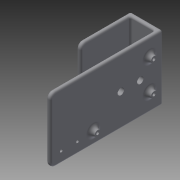
# Autodesk Inventor part: bed-stopper
Saved by Autodesk Inventor 2014 (Build 180170000, 170)
## iProperties
Created: 2017-07-21
Part Number: bed-stopper
Material: 一般
Document SubType Name: Modeling
Designer: hide
Density: 1 g/cm^3
Appearance: 既定
Author: hide
Autodesk Inventor part; units mm, degrees
ref_plane "YZ Plane" through (0, 0, 0) normal (1, 0, 0) x (0, 1, 0)
ref_plane "XZ Plane" through (0, 0, 0) normal (0, 1, 0) x (-1, 0, 0)
ref_plane "XY Plane" through (0, 0, 0) normal (0, 0, 1) x (1, 0, 0)
sketch "スケッチ1" plane through (0, 0, 0) normal (0, 0, 1) x (1, 0, 0)
  line L0 (0, -46) -> (0, 0)
  line L1 (22, 0) -> (22, -100)
  line L2 (22, -100) -> (26, -100)
  line L3 (26, -100) -> (26, 4)
  line L4 (26, 4) -> (-4, 4)
  line L5 (-4, 4) -> (-4, -46)
  line L6 (-4, -46) -> (0, -46)
  line L7 (0, 0) -> (22, 0)
  dimension "d0" = 4
  dimension "d1" = 4
  dimension "d2" = 4
  dimension "d3" = 100
  dimension "d4" = 22
  dimension "d5" = 50
  constraints: 16 end point, 6 parallel, 1 perpendicular, 1 vertical
  measures "d0" distance between parallel lines of L4 L7
  measures "d1" distance between parallel lines of L5 L0
  measures "d2" distance between parallel lines of L3 L1
  measures "d3" distance between parallel lines of L7 L2
  measures "d4" distance between parallel lines of L0 L1
  measures "d5" distance between parallel lines of L4 L6
extrude "押し出し1" add sketch "スケッチ1" along normal blind 60
sketch "スケッチ2" plane through (-4, -46, 0) normal (-1, 0, 0) x (0, 0, 1)
  line L0 (0, 0) -> (0, 50) projected
  line L1 (0, 50) -> (60, 50) projected
  line L2 (17.5, 35) -> (42.5, 35)
  line L3 (42.5, 35) -> (42.5, 6)
  line L4 (42.5, 6) -> (17.5, 6)
  line L5 (17.5, 6) -> (17.5, 35)
  point P0 (0, 46)
  dimension "d8" = 29
  dimension "d9" = 25
  dimension "d10" = 17.5
  dimension "d11" = 15
  constraints: 8 end point, 2 parallel, 1 horizontal, 1 perpendicular
  measures "d8" distance of L4.end L2.start
  measures "d9" distance of L2.start L2.end
  measures "d10" distance between parallel lines of L5 L0
  measures "d11" distance between parallel lines of L2 L1
extrude "押し出し2" add sketch "スケッチ2" along normal blind 5
fillet "フィレット1" radius 5 4 edges at (-6.5, -11, 17.5) (-6.5, -11, 42.5) (-6.5, -40, 17.5) (-6.5, -40, 42.5)
sketch "スケッチ3" plane through (-9, -46, 0) normal (-1, 0, 0) x (0, 0, 1)
  line L0 (17.5, 30) -> (17.5, 11) projected
  circle A0 centre (30, 29) radius 1.75
  circle A1 centre (30, 11) radius 1.75
  line L1 (37.5, 35) -> (22.5, 35) projected
  point P0 (0, 46)
  dimension "d15" = 3.5
  dimension "d16" = 3.5
  dimension "d17" = 0
  dimension "d18" = 18
  dimension "d19" = 12.5
  dimension "d24" = 6
  constraints: 2 centre point
  measures "d15" diameter of A0
  measures "d16" diameter of A1
  measures "d17" horizontal distance of A0.centre A1.centre
  measures "d18" distance of A1.centre A0.centre
  measures "d19" distance from line of A1.centre L0
  measures "d24" distance from line of A0.centre L1
extrude "押し出し3" cut sketch "スケッチ3" against normal blind 200
fillet "フィレット2" radius 5 4 edges at (24, -100, 0) (24, -100, 60) (-2, -46, 0) (-2, -46, 60)
fillet "フィレット3" radius 1.8 26 edges at (22, 0, 30) (0, 0, 30) (26, 4, 30) (-4, 4, 30) (-4, -44.5355, 58.5355) (-4, -18.5, 60) (-4, -44.5355, 1.4645) (-4, -18.5, 0) (-4, -46, 30) (26, -98.5355, 1.4645) (26, -100, 30) (26, -45.5, 0) (11, 4, 0) (0, -44.5355, 1.4645) (0, -46, 30) (0, -44.5355, 58.5355) (0, -20.5, 60) (0, -20.5, 0) (22, -98.5355, 1.4645) (22, -100, 30) (22, -47.5, 0) (11, 0, 0) (22, -98.5355, 58.5355) (22, -47.5, 60) (11, 4, 60) (11, 0, 60)
sketch "スケッチ4" plane through (-9, -46, 0) normal (-1, 0, 0) x (0, 0, 1)
  line L0 (17.5, 30) -> (17.5, 11) projected
  line L1 (17.5, 17) -> (33.5, 17)
  line L2 (33.5, 17) -> (33.5, 23)
  line L3 (33.5, 23) -> (17.5, 23)
  line L4 (17.5, 23) -> (17.5, 17)
  line L5 (37.5, 35) -> (22.5, 35) projected
  point P0 (0, 46)
  dimension "d25" = 6
  dimension "d35" = 12
  dimension "d36" = 16
  constraints: 8 end point, 2 parallel, 1 horizontal, 1 perpendicular, 1 point on line
  measures "d25" distance of L1.end L2.end
  measures "d35" distance between parallel lines of L5 L3
  measures "d36" distance between parallel lines of L0 L2
extrude "押し出し4" cut sketch "スケッチ4" against normal blind 5
sketch "スケッチ5" plane through (0, -41, 1.8) normal (1, 0, 0) x (0, 0, -1)
  circle A0 centre (-28.2, 6) radius 1.75 projected
  circle A1 centre (-28.2, 24) radius 1.75 projected
  circle A2 centre (-28.2, 24) radius 3
  circle A3 centre (-28.2, 6) radius 3
  point P0 (1.8, 41)
  dimension "d28" = 6
  dimension "d29" = 6
  constraints: 2 centre point, 2 coincident
  measures "d28" diameter of A2
  measures "d29" diameter of A3
extrude "押し出し5" cut sketch "スケッチ5" along normal blind 100 and the other way blind 6.5
fillet "フィレット4" radius 5 9 edges at (-4, -38.5355, 18.9645) (-4, -32, 17.5) (-4, -38.5355, 41.0355) (-4, -25.5, 42.5) (-4, -12.4645, 41.0355) (-4, -11, 30) (-4, -12.4645, 18.9645) (-4, -19.5, 17.5) (-4, -40, 30)
sketch "スケッチ6" plane through (22, -95, 58.2) normal (-1, 0, 0) x (0, 0, 1)
  circle A0 centre (-48.2, 20) radius 3
  circle A1 centre (-48.2, 5) radius 3
  line L0 (-58.2, 93.2) -> (-58.2, 0) projected
  line L1 (-53.2, -5) -> (-3.2, -5) projected
  point P0 (-58.2, 95)
  dimension "d37" = 6
  dimension "d38" = 6
  dimension "d39" = 0
  dimension "d40" = 15
  dimension "d41" = 10
  dimension "d42" = 10
  constraints: 2 centre point
  measures "d37" diameter of A0
  measures "d38" diameter of A1
  measures "d39" horizontal distance of A1.centre A0.centre
  measures "d40" distance of A0.centre A1.centre
  measures "d41" distance from line of L0 A1.centre
  measures "d42" distance from line of L1 A1.centre
extrude "押し出し6" add sketch "スケッチ6" along normal blind 4
sketch "スケッチ7" plane through (26, -95, 58.2) normal (1, 0, 0) x (0, 0, -1)
  circle A0 centre (28.2, 78) radius 3 projected
  circle A1 centre (28.2, 60) radius 3 projected
  line L0 (0, 97.2) -> (56.4, 97.2) projected
  line L1 (0, 0) -> (0, 97.2) projected
  arc A2 (0, 0) -> (3.2, -3.2) centre (3.2, 0) ccw projected
  line L2 (53.2, -3.2) -> (3.2, -3.2) projected
  arc A3 (53.2, -3.2) -> (56.4, 0) centre (53.2, 0) ccw projected
  line L3 (56.4, 97.2) -> (56.4, 0) projected
  circle A4 centre (48.2, 5) radius 3 projected
  circle A5 centre (48.2, 20) radius 3 projected
  circle A6 centre (48.2, 20) radius 1.25
  circle A7 centre (48.2, 5) radius 1.25
  point P0 (58.2, 95)
  dimension "d45" = 2.5
  dimension "d46" = 2.5
  constraints: 2 centre point, 2 coincident
  measures "d45" diameter of A6
  measures "d46" diameter of A7
extrude "押し出し7" cut sketch "スケッチ7" against normal blind 6 contours A6 | A7
fillet "フィレット5" radius 4 2 edges at (22, -90, 7) (22, -75, 7)
sketch "スケッチ8" plane through (26, -95, 58.2) normal (1, 0, 0) x (0, 0, -1)
  circle A0 centre (13.8485, 86.7115) radius 1.35
  circle A1 centre (42.0485, 86.7115) radius 1.35
  circle A2 centre (47.0485, 34.7115) radius 1.35
  point P0 (58.2, 95)
  dimension "d51" = 2.7
  dimension "d52" = 2.7
  dimension "d53" = 2.7
  dimension "d54" = 28.2
  dimension "d55" = 0
  dimension "d56" = 52
  dimension "d57" = 5
  constraints: 3 centre point
  measures "d51" diameter of A0
  measures "d52" diameter of A1
  measures "d53" diameter of A2
  measures "d54" distance of A1.centre A0.centre
  measures "d55" vertical distance of A0.centre A1.centre
  measures "d56" vertical distance of A1.centre A2.centre
  measures "d57" horizontal distance of A1.centre A2.centre
extrude "押し出し8" cut sketch "スケッチ8" against normal blind 6
sketch "スケッチ9" plane through (26, -95, 58.2) normal (1, 0, 0) x (0, 0, -1)
  circle A0 centre (42.0485, 86.7115) radius 1.35 projected
  circle A1 centre (13.8485, 86.7115) radius 1.35 projected
  circle A2 centre (47.0485, 34.7115) radius 1.35 projected
  circle A3 centre (13.8485, 86.7115) radius 2.75
  circle A4 centre (42.0485, 86.7115) radius 2.75
  circle A5 centre (47.0485, 34.7115) radius 2.75
  point P0 (58.2, 95)
  dimension "d60" = 1.4
  dimension "d61" = 1.4
  dimension "d62" = 1.4
  constraints: 3 centre point, 3 coincident
  measures "d60" radial gap between concentric circles of A1 A3
  measures "d61" radial gap between concentric circles of A4 A0
  measures "d62" radial gap between concentric circles of A5 A2
extrude "押し出し9" add sketch "スケッチ9" along normal blind 4
fillet "フィレット6" radius 4 3 edges at (26, -8.2885, 47.1015) (26, -8.2885, 18.9015) (26, -60.2885, 13.9015)
equation "\"d0\" = d2"
equation "\"d1\" = d2"
equation "\"d16\" = d15"
equation "\"d29\" = d28"
equation "\"d38\" = d37"
equation "\"d46\" = d45"
equation "\"d52\" = d51"
equation "\"d53\" = d51"
equation "\"d61\" = d60"
equation "\"d62\" = d60"
